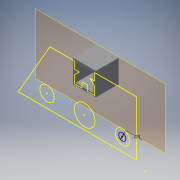
# Autodesk Inventor part: Right X End
Saved by Autodesk Inventor 2016 (Build 200138000, 138)
## iProperties
Created: 2016-04-10
Part Number: Right X End
Material: Generic
Document SubType Name: Modeling
Designer: Scott
Density: 1 g/cm^3
Appearance: Default
Author: Scott
Autodesk Inventor part; units mm, degrees
ref_plane "YZ Plane" through (0, 0, 0) normal (1, 0, 0) x (0, 1, 0)
ref_plane "XZ Plane" through (0, 0, 0) normal (0, 1, 0) x (-1, 0, 0)
ref_plane "XY Plane" through (0, 0, 0) normal (0, 0, 1) x (1, 0, 0)
ref_plane "Work Plane1" through (0, 0, 0) normal (0, 0, 1) x (1, 0, 0)
sketch "Sketch1" plane through (0, 0, 0) normal (0, 0, 1) x (1, 0, 0)
  circle A0 centre (-25.4098, 20.8167) radius 8 projected
  circle A1 centre (-109.1654, 20.8167) radius 8 projected
  circle A2 centre (-67.2876, 20.8167) radius 11.5 projected
  line L0 (-56.2876, 67.31) -> (-56.2876, 59.315) projected
  line L1 (-56.2876, 59.315) -> (-61.2876, 59.315) projected
  line L2 (-61.2876, 59.315) -> (-56.2876, 54.315) projected
  line L3 (-56.2876, 54.315) -> (-56.2876, 45.32) projected
  line L4 (-56.2876, 45.32) -> (-64.2876, 45.32) projected
  line L5 (-64.2876, 51.32) -> (-64.2876, 45.32) projected
  line L6 (-70.2876, 51.32) -> (-64.2876, 51.32) projected
  line L7 (-70.2876, 45.32) -> (-70.2876, 51.32) projected
  line L8 (-70.2876, 45.32) -> (-78.2876, 45.32) projected
  line L9 (-78.2876, 45.32) -> (-78.2876, 54.315) projected
  line L10 (-78.2876, 54.315) -> (-73.2876, 59.315) projected
  line L11 (-73.2876, 59.315) -> (-78.2876, 59.315) projected
  line L12 (-78.2876, 59.315) -> (-78.2876, 67.31) projected
  line L13 (-78.2876, 67.31) -> (-105.9385, 67.31) projected
  line L14 (-105.9385, 67.31) -> (-141.1337, 6.35) projected
  line L15 (-141.1337, 6.35) -> (-9.2697, 6.35) projected
  line L16 (-9.2697, 6.35) -> (-9.2697, 67.31) projected
  line L17 (-9.2697, 67.31) -> (-56.2876, 67.31) projected
  circle A3 centre (-109.1654, 20.8167) radius 8 projected
  circle A4 centre (-25.4098, 20.8167) radius 8 projected
  circle A5 centre (-67.2876, 20.8167) radius 11.5 projected
  line L18 (-77.2876, 46.815) -> (-57.2876, 46.815)
  line L19 (-57.2876, 46.815) -> (-57.2876, 66.815)
  line L20 (-57.2876, 66.815) -> (-77.2876, 66.815)
  line L21 (-77.2876, 66.815) -> (-77.2876, 46.815)
  line L22 (-77.2876, 46.815) -> (-57.2876, 66.815) construction
  line L23 (-57.2876, 46.815) -> (-77.2876, 66.815) construction
  line L24 (-79.9876, 69.515) -> (-54.5876, 69.515)
  line L25 (-54.5876, 69.515) -> (-54.5876, 44.115)
  line L26 (-54.5876, 44.115) -> (-79.9876, 44.115)
  line L27 (-79.9876, 44.115) -> (-79.9876, 69.515)
  line L28 (-79.9876, 69.515) -> (-54.5876, 44.115) construction
  line L29 (-54.5876, 69.515) -> (-79.9876, 44.115) construction
  point P0 (0, 0)
  point P1 (-67.2876, 56.815)
  dimension "d0" = 20
  dimension "d1" = 20
  dimension "d2" = 25.4
  dimension "d3" = 25.4
  constraints: 24 end point, 4 midpoint, 4 parallel, 2 horizontal, 2 perpendicular
  measures "d0" distance of L20.end L19.end
  measures "d1" distance of L19.end L18.end
  measures "d2" distance of L25.end L26.end
  measures "d3" distance of L24.end L25.end
extrude "Extrusion1" add sketch "Sketch1" along normal blind 25.4 contours L17 L25 L26 L27 L13 L12 L11 L21 L10 L9 L8 L7 L18 L5 L4 L3 L2 L19 L1 L0 | L0 L1 L19 L20 L21 L11 L12 L13 L27 L24 L25 L17 | L2 L3 L4 L5 L18 L19 | L7 L8 L9 L10 L21 L18
sketch "Sketch2" plane through (0, 0, 25.4) normal (0, 0, 1) x (1, 0, 0)
  line L0 (-56.2876, 67.31) -> (-56.2876, 59.315) projected
  line L1 (-56.2876, 59.315) -> (-61.2876, 59.315) projected
  line L2 (-61.2876, 59.315) -> (-56.2876, 54.315) projected
  line L3 (-56.2876, 54.315) -> (-56.2876, 45.32) projected
  line L4 (-56.2876, 45.32) -> (-64.2876, 45.32) projected
  line L5 (-64.2876, 51.32) -> (-64.2876, 45.32) projected
  line L6 (-70.2876, 51.32) -> (-64.2876, 51.32) projected
  line L7 (-70.2876, 45.32) -> (-70.2876, 51.32) projected
  line L8 (-70.2876, 45.32) -> (-78.2876, 45.32) projected
  line L9 (-78.2876, 45.32) -> (-78.2876, 54.315) projected
  line L10 (-78.2876, 54.315) -> (-73.2876, 59.315) projected
  line L11 (-73.2876, 59.315) -> (-78.2876, 59.315) projected
  line L12 (-78.2876, 59.315) -> (-78.2876, 67.31) projected
  line L13 (-78.2876, 67.31) -> (-105.9385, 67.31) projected
  line L14 (-105.9385, 67.31) -> (-141.1337, 6.35) projected
  line L15 (-141.1337, 6.35) -> (-9.2697, 6.35) projected
  line L16 (-9.2697, 6.35) -> (-9.2697, 67.31) projected
  line L17 (-9.2697, 67.31) -> (-56.2876, 67.31) projected
  circle A0 centre (-109.1654, 20.8167) radius 8 projected
  circle A1 centre (-25.4098, 20.8167) radius 8 projected
  circle A2 centre (-67.2876, 20.8167) radius 11.5 projected
  circle A3 centre (-25.4098, 20.8167) radius 4
  point P0 (0, 0)
  dimension "d6" = 8
  constraints: 1 centre point, 1 coincident
  measures "d6" diameter of A3
body "Solid1"
